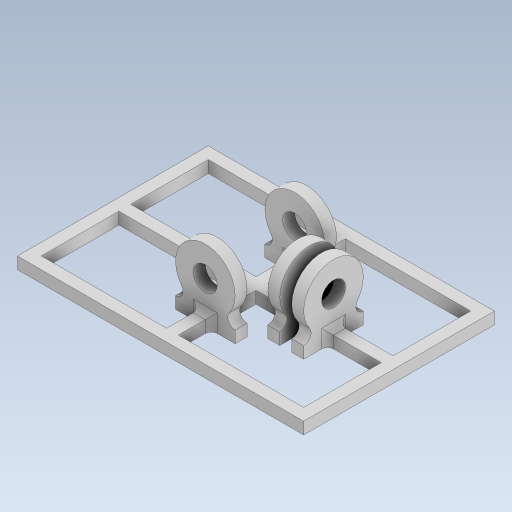
# Autodesk Inventor part: Chassis
Saved by Autodesk Inventor 2023 (Build 270158000, 158)
## iProperties
Created: 2023-02-24
Part Number: Chassis
Material: Generic
Document SubType Name: Modeling
Designer: Dave
Density: 1 g/cm^3
Appearance: Default
Author: Dave
Autodesk Inventor part; units mm, degrees
ref_plane "YZ Plane" through (0, 0, 0) normal (1, 0, 0) x (0, 1, 0)
ref_plane "XZ Plane" through (0, 0, 0) normal (0, 1, 0) x (-1, 0, 0)
ref_plane "XY Plane" through (0, 0, 0) normal (0, 0, 1) x (1, 0, 0)
sketch "Sketch1" plane through (0, 0, 0) normal (0, 1, 0) x (-1, 0, 0)
  line L0 (69.85, 44.45) -> (3.175, 44.45)
  line L1 (3.175, 44.45) -> (3.175, 3.175)
  line L2 (3.175, 3.175) -> (69.85, 3.175)
  line L3 (69.85, 3.175) -> (69.85, 44.45)
  line L4 (69.85, -3.175) -> (3.175, -3.175)
  line L5 (3.175, -3.175) -> (3.175, -44.45)
  line L6 (3.175, -44.45) -> (69.85, -44.45)
  line L7 (69.85, -44.45) -> (69.85, -3.175)
  line L8 (-3.175, 44.45) -> (-69.85, 44.45)
  line L9 (-69.85, 44.45) -> (-69.85, 3.175)
  line L10 (-69.85, 3.175) -> (-3.175, 3.175)
  line L11 (-3.175, 3.175) -> (-3.175, 44.45)
  line L12 (-3.175, -3.175) -> (-69.85, -3.175)
  line L13 (-69.85, -3.175) -> (-69.85, -44.45)
  line L14 (-69.85, -44.45) -> (-3.175, -44.45)
  line L15 (-3.175, -44.45) -> (-3.175, -3.175)
  line L16 (76.2, 50.8) -> (-76.2, 50.8)
  line L17 (-76.2, 50.8) -> (-76.2, -50.8)
  line L18 (-76.2, -50.8) -> (76.2, -50.8)
  line L19 (76.2, -50.8) -> (76.2, 50.8)
  line L20 (15.875, 26.9875) -> (-15.875, 26.9875)
  line L21 (-15.875, 26.9875) -> (-15.875, 20.6375)
  line L22 (-15.875, 20.6375) -> (15.875, 20.6375)
  line L23 (15.875, 20.6375) -> (15.875, 26.9875)
  line L24 (15.875, -20.6375) -> (-15.875, -20.6375)
  line L25 (-15.875, -20.6375) -> (-15.875, -26.9875)
  line L26 (-15.875, -26.9875) -> (15.875, -26.9875)
  line L27 (15.875, -26.9875) -> (15.875, -20.6375)
  line L28 (106.68, 0) -> (-106.68, 0) projected
  line L29 (-22.225, 15.875) -> (-28.575, 15.875)
  line L30 (-28.575, 15.875) -> (-28.575, -15.875)
  line L31 (-28.575, -15.875) -> (-22.225, -15.875)
  line L32 (-22.225, -15.875) -> (-22.225, 15.875)
  line L33 (-34.925, 15.875) -> (-41.275, 15.875)
  line L34 (-41.275, 15.875) -> (-41.275, -15.875)
  line L35 (-41.275, -15.875) -> (-34.925, -15.875)
  line L36 (-34.925, -15.875) -> (-34.925, 15.875)
  point P0 (0, 0)
  point P1 (-76.2, 0)
  point P2 (0, -50.8)
  point P3 (15.875, 23.8125)
  point P4 (3.175, 23.8125)
  point P5 (0, 20.6375)
  point P6 (3.175, 26.9875)
  point P7 (3.175, 20.6375)
  point P8 (3.175, -20.6375)
  point P9 (3.175, -26.9875)
  point P10 (-3.175, -26.9875)
  point P11 (-3.175, -20.6375)
  point P12 (-3.175, 20.6375)
  point P13 (-3.175, 26.9875)
  point P14 (-25.4, -15.875)
  point P15 (-38.1, -15.875)
  point P16 (-22.225, 0)
  point P17 (-22.225, -3.175)
  point P18 (-28.575, -3.175)
  point P19 (-41.275, 3.175)
  point P20 (-34.925, 3.175)
  point P21 (-34.925, -3.175)
  point P22 (-41.275, -3.175)
  point P23 (-28.575, 3.175)
  point P24 (-22.225, 3.175)
  dimension "d0" = 6.35
  dimension "d1" = 6.35
  dimension "d2" = 6.35
  dimension "d3" = 6.35
  dimension "d4" = 6.35
  dimension "d5" = 101.6
  dimension "d6" = 152.4
  dimension "d7" = 6.35
  dimension "d8" = 31.75
  dimension "d9" = 6.35
  dimension "d12" = 25.4
  dimension "d13" = 12.7
  constraints: 72 end point, 18 parallel, 11 point on line, 9 horizontal, 9 perpendicular, 8 midpoint, 5 equal length, 2 horizontal alignment, 2 vertical alignment, 4 other
  measures "d0" distance between parallel lines of L19 L3
  measures "d1" distance between parallel lines of L16 L0
  measures "d2" distance between parallel lines of L4 L2
  measures "d3" distance between parallel lines of L18 L6
  measures "d4" distance between parallel lines of L17 L13
  measures "d5" distance of L18.end L16.start
  measures "d6" distance of L17.end L18.end
  measures "d7" distance between parallel lines of L5 L15
  measures "d8" distance of L21.end L22.end
  measures "d9" distance of L22.end L20.start
  measures "d12" horizontal distance of point (-25.4, -15.875) point (0, 0)
  measures "d13" distance of point (-25.4, -15.875) point (-38.1, -15.875)
extrude "Extrusion1" add sketch "Sketch1" along normal blind 6.35 contours L0 L1 L20 L11 L8 L9 L10 L34 L28 L17 L16 L19 L32 L22 L2 L3 | L20 L23 L22 L1 | L1 L22 L11 L20 | L11 L22 L21 L20 | L32 L28 L30 L10 | L10 L30 L29 L32 | L30 L28 L36 L10 | L32 L12 L30 L28 | L28 L19 L18 L17 L34 L12 L13 L14 L15 L26 L5 L6 L7 L4 L24 L32 | L34 L33 L36 L10 | L10 L36 L28 L34 | L30 L12 L36 L28 | L32 L31 L30 L12 | L28 L36 L12 L34 | L12 L36 L35 L34 | L24 L5 L26 L15 | L15 L26 L25 L24 | L24 L27 L26 L5
sketch "Sketch2" plane through (3.175, 0, 26.9875) normal (0, 0, 1) x (1, 0, 0)
  line L0 (-79.375, 6.35) -> (73.025, 6.35) projected
  circle A0 centre (-3.175, 22.225) radius 6.35
  circle A1 centre (-3.175, 22.225) radius 15.875
  circle A2 centre (-19.05, 10.3188) radius 3.9688
  circle A3 centre (12.7, 10.3188) radius 3.9688
  point P0 (-3.175, 0)
  point P1 (-3.175, 6.35)
  point P2 (9.525, 12.7)
  point P3 (-15.875, 12.7)
  point P4 (-19.05, 6.35)
  point P5 (12.7, 6.35)
  dimension "d14" = 12.7
  dimension "d15" = 31.75
  dimension "d16" = 31.75
  constraints: 5 tangent, 4 centre point, 1 coincident, 1 equal radius, 1 midpoint, 1 vertical alignment
  measures "d14" diameter of A0
  measures "d15" diameter of A1
  measures "d16" distance of A2.centre A3.centre
extrude "Extrusion2" add sketch "Sketch2" against normal blind 6.35 contours A2 A1 L0 | A1 A3 L0 | A1
mirror "Mirror1" about plane through (0, 0, 0) normal (0, 0, 1) of "Extrusion2"
sketch "Sketch3" plane through (41.275, 0, -3.175) normal (1, 0, 0) x (0, 0, -1)
  line L0 (0, 0) -> (0, 6.35) projected
  circle A0 centre (-3.175, 22.225) radius 6.35
  circle A1 centre (-19.05, 10.3188) radius 3.9687
  circle A2 centre (12.7, 10.3188) radius 3.9687
  line L1 (-53.975, 6.35) -> (47.625, 6.35) projected
  circle A3 centre (-3.175, 22.225) radius 15.875
  line L2 (0, 6.35) -> (12.7, 6.35) projected
  point P0 (-3.175, 0)
  point P1 (-3.175, 6.35)
  point P2 (-3.175, 6.35)
  point P3 (12.7, 6.35)
  point P4 (9.525, 12.7)
  point P5 (-15.875, 12.7)
  point P6 (-19.05, 6.35)
  dimension "d20" = 12.7
  dimension "d22" = 31.75
  dimension "d23" = 31.75
  constraints: 3 centre point, 3 tangent, 2 midpoint, 1 coincident, 1 horizontal, 1 vertical alignment, 4 other
  measures "d20" diameter of A0
  measures "d22" distance of point (12.7, 10.319) A1.centre
  measures "d23" diameter of A3
extrude "Extrusion3" add sketch "Sketch3" against normal up to surface (6.35 mm away) contours A1 A3 L1 | A3 | A3 A2 L1
pattern_linear "Rectangular Pattern1" count 2 spacing 12.7 along (-1, 0, 0) of "Extrusion3"
fillet "Fillet1" radius 3.175 23 edges at (3.175, 3.175, 26.9875) (0, 6.35, 26.9875) (-3.175, 3.175, 26.9875) (3.175, 3.175, 20.6375) (0, 6.35, 20.6375) (-3.175, 3.175, 20.6375) (41.275, 3.175, 3.175) (41.275, 6.35, 0) (41.275, 3.175, -3.175) (34.925, 3.175, 3.175) (28.575, 3.175, -3.175) (28.575, 3.175, 3.175) (28.575, 6.35, 0) (34.925, 6.35, 0) (22.225, 3.175, -3.175) (22.225, 6.35, 0) (22.225, 3.175, 3.175) (0, 6.35, -20.6375) (-3.175, 3.175, -20.6375) (3.175, 3.175, -20.6375) (3.175, 3.175, -26.9875) (-3.175, 3.175, -26.9875) (0, 6.35, -26.9875)
equation "\"d3\" = d1"
equation "\"d4\" = d1"
equation "\"d7\" = d0"
body "Solid1"
